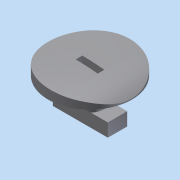
# Autodesk Inventor part: CRX brake light housing retainer
Saved by Autodesk Inventor 2011 SP2 (Build 150309200, 309)
## iProperties
Created: 2015-04-16
Part Number: CRX brake light housing retainer
Document SubType Name: Modeling
Designer: LaserMotive
Density: 1 g/cm^3
Author: LaserMotive
Autodesk Inventor part; units mm, degrees
ref_plane "YZ Plane" through (0, 0, 0) normal (1, 0, 0) x (0, 1, 0)
ref_plane "XZ Plane" through (0, 0, 0) normal (0, 1, 0) x (-1, 0, 0)
ref_plane "XY Plane" through (0, 0, 0) normal (0, 0, 1) x (1, 0, 0)
sketch "Sketch1" plane through (0, 0, 0) normal (0, 0, 1) x (1, 0, 0)
  circle A0 centre (0, 0) radius 9.5
  line L0 (-2.5, 0.75) -> (2.5, 0.75)
  line L1 (2.5, 0.75) -> (2.5, -0.75)
  line L2 (2.5, -0.75) -> (-2.5, -0.75)
  line L3 (-2.5, -0.75) -> (-2.5, 0.75)
  line L4 (0, -0.75) -> (0, 0.75) construction
  line L5 (0, -13.3) -> (0, 13.3) construction
  line L6 (-13.3, 0) -> (13.3, 0) construction
  point P0 (2.5, 0)
  dimension "d0" = 19
  dimension "d1" = 1.5
  dimension "d2" = 5
  constraints: 10 end point, 4 midpoint, 2 coincident, 2 parallel, 2 point on line, 1 centre point, 1 horizontal, 1 perpendicular
  measures "d0" diameter of A0
  measures "d1" distance of L0.end L1.end
  measures "d2" distance of L0.start L0.end
extrude "Extrusion1" add sketch "Sketch1" along normal blind 2.3
sketch "Sketch2" plane through (0, 0, 0) normal (0, 1, 0) x (-1, 0, 0)
  line L0 (-2.5, 2.3) -> (2.5, 2.3) construction
  line L1 (2.5, 2.3) -> (-2.5, 2.3) construction
  line L2 (-9.5, 2.3) -> (9.5, 2.3) construction
  line L3 (-9.5, 2.3) -> (9.5, 2.3) construction
  line L4 (-2.5, 0) -> (2.5, 0) construction
  line L5 (2.5, 0) -> (-2.5, 0) construction
  line L6 (-9.5, 0) -> (9.5, 0) construction
  line L7 (-9.5, 0) -> (-9.5, 0.2)
  line L8 (-9.5, 0) -> (9.5, 0)
  line L9 (9.5, 0) -> (9.5, 1.9)
  arc A0 (-5.5, 1.6114) -> (-9.5, 0.2) centre (-3.57, -10.2324) ccw
  arc A1 (17.6587, 0.2303) -> (-5.5, 1.6114) centre (3.0073, -50.5943) ccw
  point P0 (0, 0)
  dimension "d5" = 12
  dimension "d6" = 0.2
  dimension "d8" = 1.9
  dimension "d9" = 4
  constraints: 6 end point, 5 point on circle, 2 centre point, 2 perpendicular, 2 tangent, 1 collinear
  measures "d5" radius of A0
  measures "d6" distance of L6.start L7.end
  measures "d8" distance of L6.end L9.end
  measures "d9" horizontal distance of L7.end A0.start
extrude "Extrusion2" cut sketch "Sketch2" along normal through all both and the other way through all keep common part
sketch "Sketch3" plane through (0, 0, 0) normal (0, 1, 0) x (-1, 0, 0)
  line L0 (-2.5, 0) -> (2.5, 0) construction
  line L1 (2.5, 0) -> (-2.5, 0) construction
  line L2 (-9.5, 0) -> (9.5, 0) construction
  line L3 (-3.25, 0) -> (0, 0)
  line L4 (0, 0) -> (0, -5)
  line L5 (0, -5) -> (-3.25, -5)
  line L6 (-3.25, -5) -> (-3.25, 0)
  point P0 (0, 0)
  dimension "d12" = 3.25
  dimension "d13" = 5
  constraints: 8 end point, 3 midpoint, 2 parallel, 1 horizontal, 1 perpendicular, 1 point on line
  measures "d12" distance of L4.end L5.end
  measures "d13" distance of L5.end L3.start
revolve "Revolution1" add sketch "Sketch3" angle 360 about axis through (0, 0, 0) along (0, 0, -1)
sketch "Sketch4" plane through (0, 0, 0) normal (0, 1, 0) x (-1, 0, 0)
  line L0 (-6.25, -5) -> (6.25, -5)
  line L1 (6.25, -5) -> (6.25, -8)
  line L2 (6.25, -8) -> (-6.25, -8)
  line L3 (-6.25, -8) -> (-6.25, -5)
  line L4 (0, -12.0667) -> (0, 4.6989) construction
  line L5 (3.25, -5) -> (-3.25, -5) construction
  point P0 (0, 0)
  point P1 (0, -5)
  dimension "d16" = 3
  dimension "d17" = 12.5
  constraints: 8 end point, 2 midpoint, 2 parallel, 1 horizontal, 1 perpendicular
  measures "d16" distance between parallel lines of L2 L0
  measures "d17" distance between parallel lines of L1 L3
extrude "Extrusion3" add sketch "Sketch4" along normal blind 2.2 and the other way blind 2.2
sketch "Sketch5" plane through (0, 0, 0) normal (1, 0, 0) x (0, 1, 0)
  line L0 (2.2, -5) -> (2.2, -8) construction
  line L1 (2.2, -8) -> (2.2, -5) construction
  line L2 (3.25, -5) -> (3.25, 0) construction
  line L3 (-3.25, -5) -> (-3.25, 0) construction
  line L4 (-2.2, -5) -> (-2.2, -8) construction
  line L5 (-2.2, -8) -> (-2.2, -5) construction
  line L6 (-2.2, -5) -> (-3.25, -4)
  line L7 (2.2, -5) -> (3.25, -4)
  line L8 (3.25, -4) -> (-3.25, -4)
  line L9 (-2.2, -5) -> (-3.25, -5)
  line L10 (-3.25, -5) -> (-3.25, -4)
  line L11 (2.2, -5) -> (3.25, -5)
  line L12 (3.25, -4) -> (3.25, -5)
  point P0 (0, 0)
  point P1 (2.2, -5)
  point P2 (2.2, -5)
  dimension "d23" = 1
  constraints: 14 end point, 3 perpendicular, 2 point on line, 1 collinear, 1 parallel
  measures "d23" distance of L7.end L2.start
extrude "Extrusion4" cut sketch "Sketch5" along normal through all both and the other way through all
body "Solid1"
